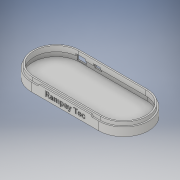
# Autodesk Inventor part: Base inspirómetro
Saved by Autodesk Inventor 2019 (Build 230136000, 136)
## iProperties
Created: 2020-12-03
Part Number: Base inspirómetro
Material: Generic
Document SubType Name: Modeling
Designer: Abraham
Density: 1 g/cm^3
Appearance: Default
Author: Abraham
Autodesk Inventor part; units mm, degrees
note: some values were not read from the file. Chosen so that the rebuilt part matches the saved one: direction of "Emboss1".
ref_plane "YZ Plane" through (0, 0, 0) normal (1, 0, 0) x (0, 1, 0)
ref_plane "XZ Plane" through (0, 0, 0) normal (0, 1, 0) x (-1, 0, 0)
ref_plane "XY Plane" through (0, 0, 0) normal (0, 0, 1) x (1, 0, 0)
sketch "Sketch1" plane through (0, 0, 0) normal (0, 1, 0) x (-1, 0, 0)
  line L0 (-43, 35.5) -> (53, 35.5)
  arc A0 (53, -35.5) -> (53, 35.5) centre (53, 0) ccw
  arc A1 (-43, 35.5) -> (-43, -35.5) centre (-43, 0) ccw
  line L1 (53, -35.5) -> (-43, -35.5)
  point P0 (0, 0)
  constraints: 4 end point, 4 point on circle, 2 centre point
extrude "Extrusion1" add sketch "Sketch1" against normal blind 2
sketch "Sketch2" plane through (0, 0, 0) normal (0, 1, 0) x (1, 0, 0)
  arc A0 (43, -35.5) -> (43, 35.5) centre (43, 0) ccw projected
  arc A1 (43, -35.5) -> (43, 35.5) centre (43, 0) ccw
  line L0 (43, 35.5) -> (-53, 35.5)
  line L1 (43, -35.5) -> (-53, -35.5)
  line L2 (-53, 35.5) -> (43, 35.5) projected
  line L3 (43, -35.5) -> (-53, -35.5) projected
  arc A2 (-53, 35.5) -> (-53, -35.5) centre (-53, 0) ccw
  line L4 (-53, 33.5) -> (43, 33.5)
  arc A3 (43, -33.5) -> (43, 33.5) centre (43, 0) ccw
  line L5 (43, -33.5) -> (-53, -33.5)
  arc A4 (-53, 33.5) -> (-53, -33.5) centre (-53, 0) ccw
  point P0 (0, 0)
  constraints: 8 end point, 8 point on circle, 4 centre point, 3 other
extrude "Extrusion2" add sketch "Sketch2" along normal blind 10
sketch "Sketch3" plane through (0, 10, 0) normal (0, 1, 0) x (1, 0, 0)
  line L0 (-43.5, 33.5) -> (-43.5, 35.5)
  line L1 (-43.5, -33.5) -> (-43.5, -35.5)
  line L2 (33.615, -33.5) -> (33.615, -35.5)
  line L3 (33.615, 33.5) -> (33.615, 35.5)
  line L4 (31.615, 33.5) -> (31.615, 35.5)
  line L5 (-41.5, 33.5) -> (-41.5, 35.5)
  line L6 (-41.5, -33.5) -> (-41.5, -35.5)
  line L7 (31.615, -33.5) -> (31.615, -35.5)
  line L8 (31.615, -33.5) -> (-41.5, -33.5)
  line L9 (-41.5, -35.5) -> (31.615, -35.5)
  line L10 (31.615, 35.5) -> (-41.5, 35.5)
  line L11 (-41.5, 33.5) -> (31.615, 33.5)
  point P0 (0, 0)
  dimension "d10" = 2
  dimension "d11" = 2
  dimension "d12" = 2
  dimension "d13" = 2
  constraints: 24 end point, 4 parallel, 3 vertical
  measures "d10" distance between parallel lines of L3 L4
  measures "d11" distance between parallel lines of L0 L5
  measures "d12" distance between parallel lines of L1 L6
  measures "d13" distance between parallel lines of L2 L7
extrude "Extrusion3" add sketch "Sketch3" along normal blind 2.5
sketch "Sketch4" plane through (-53, -2, 35.5) normal (0, 0, 1) x (1, 0, 0)
  line L0 (11.5, 12) -> (9.5, 12)
  line L1 (11.5, 12) -> (11.5, 14.5) projected
  line L2 (11.5, 12) -> (11.5, 14.5)
  line L3 (9.5, 12) -> (11.5, 14.5)
  line L4 (84.615, 12) -> (84.615, 14.5) projected
  line L5 (84.615, 12) -> (86.615, 12)
  line L6 (84.615, 14.5) -> (86.615, 12)
  point P0 (53, 2)
  dimension "d16" = 2
  dimension "d17" = 2
  constraints: 10 end point, 1 vertical
  measures "d16" distance of L0.start L0.end
  measures "d17" distance of L4.start L5.end
extrude "Extrusion4" add sketch "Sketch4" against normal blind 2
sketch "Sketch5" plane through (43, -2, -35.5) normal (0, 0, -1) x (-1, 0, 0)
  line L0 (11.385, 14.5) -> (84.5, 14.5) projected
  line L1 (84.5, 12) -> (96, 12) projected
  line L2 (84.5, 14.5) -> (84.5, 12)
  line L3 (84.5, 12) -> (86.5, 12)
  line L4 (86.5, 12) -> (84.5, 14.5)
  line L5 (11.385, 12) -> (9.385, 12)
  line L6 (11.385, 12) -> (0, 12) projected
  line L7 (11.385, 14.5) -> (9.385, 12) projected
  line L8 (9.385, 12) -> (11.385, 14.5)
  line L9 (11.385, 12) -> (11.385, 14.5) projected
  line L10 (11.385, 14.5) -> (11.385, 12)
  point P0 (43, 2)
  dimension "d20" = 2
  dimension "d21" = 2
  constraints: 12 end point, 2 collinear, 2 point on line, 1 perpendicular
  measures "d20" distance of L1.start L3.end
  measures "d21" distance of L5.start L5.end
extrude "Extrusion5" add sketch "Sketch5" against normal blind 2
sketch "Sketch6" plane through (0, 10, 0) normal (0, 1, 0) x (1, 0, 0)
  arc A0 (43, -33.5) -> (43, 33.5) centre (43, 0) ccw projected
  arc A1 (43, -33.5) -> (43, 33.5) centre (43, 0) ccw
  arc A2 (43, -35.5) -> (43, 35.5) centre (43, 0) ccw projected
  line L0 (-53, 33.5) -> (-43.5, 33.5) projected
  arc A3 (-53, 33.5) -> (-53, -33.5) centre (-53, 0) ccw projected
  arc A4 (-53, 33.5) -> (-53, -33.5) centre (-53, 0) ccw
  line L1 (-53, 33.5) -> (43, 33.5)
  line L2 (-43.5, -33.5) -> (-53, -33.5) projected
  line L3 (-53, -33.5) -> (43, -33.5)
  arc A5 (43, -31.5) -> (43, 31.5) centre (43, 0) ccw
  line L4 (43, -31.5) -> (-53, -31.5)
  arc A6 (-53, 31.5) -> (-53, -31.5) centre (-53, 0) ccw
  line L5 (-53, 31.5) -> (43, 31.5)
  point P0 (0, 0)
  constraints: 8 end point, 8 point on circle, 4 centre point, 1 collinear, 1 concentric, 1 horizontal, 3 other
extrude "Extrusion6" add sketch "Sketch6" against normal blind 2.5 and the other way blind 5
sketch "Sketch8" plane through (43, -2, -35.5) normal (0, 0, -1) x (-1, 0, 0)
  line L0 (86.5, 12) -> (99.5, 12)
  line L1 (84.5, 14.5) -> (11.385, 14.5) projected
  line L2 (99.5, 12) -> (99.5, 3)
  line L3 (129.5, 2) -> (96, 2) projected
  line L4 (99.5, 3) -> (86.5, 3)
  line L5 (86.5, 3) -> (86.5, 12)
  line L6 (74.5, 12) -> (74.5, 6)
  line L7 (74.5, 6) -> (64.5, 6)
  line L8 (64.5, 6) -> (64.5, 12)
  line L9 (64.5, 12) -> (74.5, 12)
  point P0 (43, 2)
  constraints: 16 end point, 3 perpendicular, 2 parallel
extrude "Extrusion7" cut sketch "Sketch8" against normal blind 5
sketch "Sketch9" plane through (-53, -2, 35.5) normal (0, 0, 1) x (1, 0, 0)
  line L0 (11.4147, 12.1537) -> (84.7333, 12.1537) construction
  line L1 (84.7333, 12.1537) -> (84.7333, 1.7272) construction
  line L2 (84.7333, 1.7272) -> (11.4147, 1.7272) construction
  line L3 (11.4147, 1.7272) -> (11.4147, 12.1537) construction
  line L4 (19.9833, 4.4702) -> (19.9833, 11.4702)
  line L5 (19.9833, 11.4702) -> (22.9605, 11.4702)
  spline S0 degree 2 poles (22.9605, 11.4702) (24.0862, 11.4702) (25.1, 11.0914) (25.7135, 10.131) (25.7135, 9.5068) knots 0 0 0 1 2 3 3 3
  spline S1 degree 2 poles (25.7135, 9.5068) (25.7135, 8.7225) (24.7905, 7.6928) (23.8675, 7.5594) knots 0 0 0 1 2 2 2
  spline S2 degree 2 poles (23.8675, 7.5594) (24.3263, 7.2926) (24.9239, 6.6524) (25.4308, 5.8361) knots 0 0 0 1 2 2 2
  line L6 (25.4308, 5.8361) -> (26.2844, 4.4702)
  line L7 (26.2844, 4.4702) -> (24.5931, 4.4702)
  line L8 (24.5931, 4.4702) -> (23.574, 5.9961)
  spline S3 degree 2 poles (23.574, 5.9961) (23.0245, 6.8124) (22.6243, 7.2393) (22.1762, 7.394) (21.6853, 7.394) knots 0 0 0 1 2 3 3 3
  line L9 (21.6853, 7.394) -> (21.3972, 7.394)
  line L10 (21.3972, 7.394) -> (21.3972, 4.4702)
  line L11 (21.3972, 4.4702) -> (19.9833, 4.4702)
  line L12 (21.3972, 8.5091) -> (22.4429, 8.5091)
  spline S4 degree 2 poles (22.4429, 8.5091) (23.462, 8.5091) (23.9689, 8.6798) (24.257, 9.1013) (24.257, 9.4161) knots 0 0 0 1 2 3 3 3
  spline S5 degree 2 poles (24.257, 9.4161) (24.257, 9.7682) (23.8782, 10.2057) (23.5367, 10.2644) knots 0 0 0 1 2 2 2
  spline S6 degree 2 poles (23.5367, 10.2644) (23.3606, 10.2857) (22.5016, 10.2857) knots 0 0 0 1 1 1
  line L13 (22.5016, 10.2857) -> (21.3972, 10.2857)
  line L14 (21.3972, 10.2857) -> (21.3972, 8.5091)
  line L15 (28.0344, 7.9969) -> (26.8179, 8.2156)
  spline S7 degree 2 poles (26.8179, 8.2156) (27.026, 8.9519) (28.0291, 9.6562) (29.0161, 9.6562) knots 0 0 0 1 2 2 2
  spline S8 degree 2 poles (29.0161, 9.6562) (29.9178, 9.6562) (30.7981, 9.2293) (31.1556, 8.5784) (31.1556, 7.7034) knots 0 0 0 1 2 3 3 3
  line L16 (31.1556, 7.7034) -> (31.1343, 6.1348)
  spline S9 degree 2 poles (31.1343, 6.1348) (31.1343, 5.4679) (31.2623, 4.833) (31.4384, 4.4702) knots 0 0 0 1 2 2 2
  line L17 (31.4384, 4.4702) -> (30.1099, 4.4702)
  spline S10 degree 2 poles (30.1099, 4.4702) (30.0565, 4.6036) (29.9818, 4.865) knots 0 0 0 1 1 1
  spline S11 degree 2 poles (29.9818, 4.865) (29.9498, 4.9877) (29.9338, 5.0251) knots 0 0 0 1 1 1
  spline S12 degree 2 poles (29.9338, 5.0251) (29.5923, 4.6943) (28.808, 4.3582) (28.3652, 4.3582) knots 0 0 0 1 2 2 2
  spline S13 degree 2 poles (28.3652, 4.3582) (27.5809, 4.3582) (26.6792, 5.2065) (26.6792, 5.8574) knots 0 0 0 1 2 2 2
  spline S14 degree 2 poles (26.6792, 5.8574) (26.6792, 6.2896) (27.09, 6.9618) (27.8317, 7.3193) (28.5306, 7.4527) knots 0 0 0 1 2 3 3 3
  spline S15 degree 2 poles (28.5306, 7.4527) (29.4696, 7.6287) (29.8324, 7.7835) knots 0 0 0 1 1 1
  line L18 (29.8324, 7.7835) -> (29.8324, 7.9168)
  spline S16 degree 2 poles (29.8324, 7.9168) (29.8324, 8.301) (29.4483, 8.6318) (28.9201, 8.6318) knots 0 0 0 1 2 2 2
  spline S17 degree 2 poles (28.9201, 8.6318) (28.5626, 8.6318) (28.1571, 8.349) (28.0344, 7.9969) knots 0 0 0 1 2 2 2
  spline S18 degree 2 poles (29.8324, 6.9085) (29.5763, 6.8231) (28.4559, 6.583) (28.2852, 6.471) knots 0 0 0 1 2 2 2
  spline S19 degree 2 poles (28.2852, 6.471) (28.0237, 6.2842) (28.0237, 5.9961) knots 0 0 0 1 1 1
  spline S20 degree 2 poles (28.0237, 5.9961) (28.0237, 5.7133) (28.4452, 5.3025) (28.7707, 5.3025) knots 0 0 0 1 2 2 2
  spline S21 degree 2 poles (28.7707, 5.3025) (29.1335, 5.3025) (29.459, 5.5426) knots 0 0 0 1 1 1
  spline S22 degree 2 poles (29.459, 5.5426) (29.7044, 5.724) (29.7791, 5.9854) knots 0 0 0 1 1 1
  spline S23 degree 2 poles (29.7791, 5.9854) (29.8324, 6.1562) (29.8324, 6.6417) knots 0 0 0 1 1 1
  line L19 (29.8324, 6.6417) -> (29.8324, 6.9085)
  line L20 (32.3721, 9.5441) -> (33.6099, 9.5441)
  line L21 (33.6099, 9.5441) -> (33.6099, 8.8505)
  spline S24 degree 2 poles (33.6099, 8.8505) (34.2768, 9.6562) (35.1945, 9.6562) knots 0 0 0 1 1 1
  spline S25 degree 2 poles (35.1945, 9.6562) (35.68, 9.6562) (36.3949, 9.256) (36.6243, 8.8505) knots 0 0 0 1 2 2 2
  spline S26 degree 2 poles (36.6243, 8.8505) (36.9605, 9.256) (37.7341, 9.6562) (38.1716, 9.6562) knots 0 0 0 1 2 2 2
  spline S27 degree 2 poles (38.1716, 9.6562) (38.7318, 9.6562) (39.5054, 9.2027) (39.6975, 8.7652) knots 0 0 0 1 2 2 2
  spline S28 degree 2 poles (39.6975, 8.7652) (39.8362, 8.4397) (39.8362, 7.7141) knots 0 0 0 1 1 1
  line L22 (39.8362, 7.7141) -> (39.8362, 4.4702)
  line L23 (39.8362, 4.4702) -> (38.4917, 4.4702)
  line L24 (38.4917, 4.4702) -> (38.4917, 7.3726)
  spline S29 degree 2 poles (38.4917, 7.3726) (38.4917, 8.1249) (38.353, 8.3437) knots 0 0 0 1 1 1
  spline S30 degree 2 poles (38.353, 8.3437) (38.1663, 8.6318) (37.7821, 8.6318) knots 0 0 0 1 1 1
  spline S31 degree 2 poles (37.7821, 8.6318) (37.4993, 8.6318) (37.0032, 8.2903) (36.7844, 7.6234) (36.7844, 6.9085) knots 0 0 0 1 2 3 3 3
  line L25 (36.7844, 6.9085) -> (36.7844, 4.4702)
  line L26 (36.7844, 4.4702) -> (35.4399, 4.4702)
  line L27 (35.4399, 4.4702) -> (35.4399, 7.2499)
  spline S32 degree 2 poles (35.4399, 7.2499) (35.4399, 7.9915) (35.2958, 8.4237) (34.9971, 8.6318) (34.7356, 8.6318) knots 0 0 0 1 2 3 3 3
  spline S33 degree 2 poles (34.7356, 8.6318) (34.4262, 8.6318) (33.93, 8.2957) (33.7166, 7.6661) (33.7166, 6.9351) knots 0 0 0 1 2 3 3 3
  line L28 (33.7166, 6.9351) -> (33.7166, 4.4702)
  line L29 (33.7166, 4.4702) -> (32.3721, 4.4702)
  line L30 (32.3721, 4.4702) -> (32.3721, 9.5441)
  line L31 (41.1274, 9.5441) -> (42.3812, 9.5441)
  line L32 (42.3812, 9.5441) -> (42.3812, 8.7972)
  spline S34 degree 2 poles (42.3812, 8.7972) (42.6266, 9.1813) (43.4536, 9.6562) (43.9605, 9.6562) knots 0 0 0 1 2 2 2
  spline S35 degree 2 poles (43.9605, 9.6562) (44.8461, 9.6562) (46.0786, 8.2743) (46.0786, 7.0365) knots 0 0 0 1 2 2 2
  spline S36 degree 2 poles (46.0786, 7.0365) (46.0786, 5.7667) (44.8355, 4.3582) (43.9551, 4.3582) knots 0 0 0 1 2 2 2
  spline S37 degree 2 poles (43.9551, 4.3582) (43.5336, 4.3582) (42.8507, 4.6943) (42.4719, 5.0998) knots 0 0 0 1 2 2 2
  line L33 (42.4719, 5.0998) -> (42.4719, 2.5388)
  line L34 (42.4719, 2.5388) -> (41.1274, 2.5388)
  line L35 (41.1274, 2.5388) -> (41.1274, 9.5441)
  spline S38 degree 2 poles (42.4506, 7.0952) (42.4506, 6.2415) (43.1335, 5.4252) (43.619, 5.4252) knots 0 0 0 1 2 2 2
  spline S39 degree 2 poles (43.619, 5.4252) (44.0885, 5.4252) (44.7128, 6.1722) (44.7128, 7.0258) knots 0 0 0 1 2 2 2
  spline S40 degree 2 poles (44.7128, 7.0258) (44.7128, 7.8208) (44.0725, 8.5944) (43.5977, 8.5944) knots 0 0 0 1 2 2 2
  spline S41 degree 2 poles (43.5977, 8.5944) (43.1015, 8.5944) (42.4506, 7.8368) (42.4506, 7.0952) knots 0 0 0 1 2 2 2
  line L36 (48.1434, 7.9969) -> (46.9269, 8.2156)
  spline S42 degree 2 poles (46.9269, 8.2156) (47.135, 8.9519) (48.1381, 9.6562) (49.1251, 9.6562) knots 0 0 0 1 2 2 2
  spline S43 degree 2 poles (49.1251, 9.6562) (50.0268, 9.6562) (50.9071, 9.2293) (51.2646, 8.5784) (51.2646, 7.7034) knots 0 0 0 1 2 3 3 3
  line L37 (51.2646, 7.7034) -> (51.2432, 6.1348)
  spline S44 degree 2 poles (51.2432, 6.1348) (51.2432, 5.4679) (51.3713, 4.833) (51.5474, 4.4702) knots 0 0 0 1 2 2 2
  line L38 (51.5474, 4.4702) -> (50.2189, 4.4702)
  spline S45 degree 2 poles (50.2189, 4.4702) (50.1655, 4.6036) (50.0908, 4.865) knots 0 0 0 1 1 1
  spline S46 degree 2 poles (50.0908, 4.865) (50.0588, 4.9877) (50.0428, 5.0251) knots 0 0 0 1 1 1
  spline S47 degree 2 poles (50.0428, 5.0251) (49.7013, 4.6943) (48.917, 4.3582) (48.4742, 4.3582) knots 0 0 0 1 2 2 2
  spline S48 degree 2 poles (48.4742, 4.3582) (47.6899, 4.3582) (46.7882, 5.2065) (46.7882, 5.8574) knots 0 0 0 1 2 2 2
  spline S49 degree 2 poles (46.7882, 5.8574) (46.7882, 6.2896) (47.199, 6.9618) (47.9407, 7.3193) (48.6396, 7.4527) knots 0 0 0 1 2 3 3 3
  spline S50 degree 2 poles (48.6396, 7.4527) (49.5786, 7.6287) (49.9414, 7.7835) knots 0 0 0 1 1 1
  line L39 (49.9414, 7.7835) -> (49.9414, 7.9168)
  spline S51 degree 2 poles (49.9414, 7.9168) (49.9414, 8.301) (49.5573, 8.6318) (49.0291, 8.6318) knots 0 0 0 1 2 2 2
  spline S52 degree 2 poles (49.0291, 8.6318) (48.6716, 8.6318) (48.2661, 8.349) (48.1434, 7.9969) knots 0 0 0 1 2 2 2
  spline S53 degree 2 poles (49.9414, 6.9085) (49.6853, 6.8231) (48.5649, 6.583) (48.3942, 6.471) knots 0 0 0 1 2 2 2
  spline S54 degree 2 poles (48.3942, 6.471) (48.1327, 6.2842) (48.1327, 5.9961) knots 0 0 0 1 1 1
  spline S55 degree 2 poles (48.1327, 5.9961) (48.1327, 5.7133) (48.5542, 5.3025) (48.8797, 5.3025) knots 0 0 0 1 2 2 2
  spline S56 degree 2 poles (48.8797, 5.3025) (49.2425, 5.3025) (49.5679, 5.5426) knots 0 0 0 1 1 1
  spline S57 degree 2 poles (49.5679, 5.5426) (49.8134, 5.724) (49.8881, 5.9854) knots 0 0 0 1 1 1
  spline S58 degree 2 poles (49.8881, 5.9854) (49.9414, 6.1562) (49.9414, 6.6417) knots 0 0 0 1 1 1
  line L40 (49.9414, 6.6417) -> (49.9414, 6.9085)
  line L41 (51.9475, 9.5441) -> (53.3774, 9.5441)
  line L42 (53.3774, 9.5441) -> (54.5939, 5.9428)
  line L43 (54.5939, 5.9428) -> (55.773, 9.5441)
  line L44 (55.773, 9.5441) -> (57.1602, 9.5441)
  line L45 (57.1602, 9.5441) -> (55.3782, 4.6569)
  line L46 (55.3782, 4.6569) -> (55.0527, 3.7766)
  spline S59 degree 2 poles (55.0527, 3.7766) (54.8766, 3.3338) (54.5565, 2.8643) (54.1404, 2.5708) (53.5321, 2.4107) (53.148, 2.4107) knots 0 0 0 1 2 3 4 4 4
  spline S60 degree 2 poles (53.148, 2.4107) (52.7638, 2.4107) (52.3904, 2.4908) knots 0 0 0 1 1 1
  line L47 (52.3904, 2.4908) -> (52.273, 3.5418)
  spline S61 degree 2 poles (52.273, 3.5418) (52.5878, 3.4778) (52.8439, 3.4778) knots 0 0 0 1 1 1
  spline S62 degree 2 poles (52.8439, 3.4778) (53.308, 3.4778) (53.7615, 4.0274) (53.8789, 4.4542) knots 0 0 0 1 2 2 2
  line L48 (53.8789, 4.4542) -> (51.9475, 9.5441)
  line L49 (62.3195, 4.4702) -> (62.3195, 10.2857)
  line L50 (62.3195, 10.2857) -> (60.244, 10.2857)
  line L51 (60.244, 10.2857) -> (60.244, 11.4702)
  line L52 (60.244, 11.4702) -> (65.8035, 11.4702)
  line L53 (65.8035, 11.4702) -> (65.8035, 10.2857)
  line L54 (65.8035, 10.2857) -> (63.7333, 10.2857)
  line L55 (63.7333, 10.2857) -> (63.7333, 4.4702)
  line L56 (63.7333, 4.4702) -> (62.3195, 4.4702)
  line L57 (69.6449, 6.0868) -> (70.9841, 5.8627)
  spline S63 degree 2 poles (70.9841, 5.8627) (70.728, 5.1264) (69.6129, 4.3582) (68.7753, 4.3582) knots 0 0 0 1 2 2 2
  spline S64 degree 2 poles (68.7753, 4.3582) (67.4521, 4.3582) (66.8172, 5.2225) knots 0 0 0 1 1 1
  spline S65 degree 2 poles (66.8172, 5.2225) (66.3157, 5.9161) (66.3157, 6.9672) knots 0 0 0 1 1 1
  spline S66 degree 2 poles (66.3157, 6.9672) (66.3157, 8.2316) (67.6335, 9.6562) (68.6419, 9.6562) knots 0 0 0 1 2 2 2
  spline S67 degree 2 poles (68.6419, 9.6562) (69.773, 9.6562) (71.0801, 8.1623) (71.0535, 6.6204) knots 0 0 0 1 2 2 2
  line L58 (71.0535, 6.6204) -> (67.6922, 6.6204)
  spline S68 degree 2 poles (67.6922, 6.6204) (67.7082, 6.0228) (68.3271, 5.3612) (68.7913, 5.3612) knots 0 0 0 1 2 2 2
  spline S69 degree 2 poles (68.7913, 5.3612) (69.1061, 5.3612) (69.5329, 5.7027) (69.6449, 6.0868) knots 0 0 0 1 2 2 2
  spline S70 degree 2 poles (69.7196, 7.442) (69.7036, 8.0236) (69.1327, 8.6318) (68.7219, 8.6318) knots 0 0 0 1 2 2 2
  spline S71 degree 2 poles (68.7219, 8.6318) (68.2844, 8.6318) (67.9963, 8.3117) knots 0 0 0 1 1 1
  spline S72 degree 2 poles (67.9963, 8.3117) (67.7135, 7.9915) (67.7135, 7.442) knots 0 0 0 1 1 1
  line L59 (67.7135, 7.442) -> (69.7196, 7.442)
  line L60 (76.5596, 8.0449) -> (75.2364, 7.8048)
  spline S73 degree 2 poles (75.2364, 7.8048) (75.1724, 8.1996) (74.6975, 8.5998) (74.3187, 8.5998) knots 0 0 0 1 2 2 2
  spline S74 degree 2 poles (74.3187, 8.5998) (73.8225, 8.5998) (73.225, 7.9062) (73.225, 7.0952) knots 0 0 0 1 2 2 2
  spline S75 degree 2 poles (73.225, 7.0952) (73.225, 6.1935) (73.8332, 5.4519) (74.34, 5.4519) knots 0 0 0 1 2 2 2
  spline S76 degree 2 poles (74.34, 5.4519) (74.7242, 5.4519) (75.2097, 5.8894) (75.3111, 6.4176) knots 0 0 0 1 2 2 2
  line L61 (75.3111, 6.4176) -> (76.6289, 6.1935)
  spline S77 degree 2 poles (76.6289, 6.1935) (76.4262, 5.2865) (75.2577, 4.3582) (74.2814, 4.3582) knots 0 0 0 1 2 2 2
  spline S78 degree 2 poles (74.2814, 4.3582) (73.1716, 4.3582) (71.8484, 5.7614) (71.8484, 7.0045) knots 0 0 0 1 2 2 2
  spline S79 degree 2 poles (71.8484, 7.0045) (71.8484, 8.2583) (73.1716, 9.6562) (74.3027, 9.6562) knots 0 0 0 1 2 2 2
  spline S80 degree 2 poles (74.3027, 9.6562) (75.2311, 9.6562) (76.3195, 8.8612) (76.5596, 8.0449) knots 0 0 0 1 2 2 2
  point P0 (53, 2)
  constraints: 2 other
emboss "Emboss1" sketch "Sketch9" operation cut depth 1 direction (0, 0, -1)
body "Solid1"
